Autodesk Fusion 360 part; units mm, degrees
(part 2 of 2)
sketch "Sketch23" plane through (0, 5, 0) normal (0, 1, 0) x (-1, 0, 0)
  circle A0 centre (-181.5, -92.25) radius 5
  circle A1 centre (-181.5, -115.25) radius 5
  circle A2 centre (-154.5, -126.75) radius 5
  circle A3 centre (-154.5, -103.75) radius 5
  circle A4 centre (-186.75, -72.25) radius 4
  circle A5 centre (-140.75, -72.25) radius 4
  circle A6 centre (-94.75, -72.25) radius 4
  circle A7 centre (-48.75, -72.25) radius 4
  circle A8 centre (-190, -170) radius 3.75
  circle A9 centre (-13.25, -72.25) radius 4
  circle A10 centre (-59.25, -72.25) radius 4
  circle A11 centre (-105.25, -72.25) radius 4
  circle A12 centre (-151.25, -72.25) radius 4
  circle A13 centre (-154.5, -92.25) radius 5
  circle A14 centre (-154.5, -115.25) radius 5
  circle A15 centre (-181.5, -126.75) radius 5
  circle A16 centre (-181.5, -103.75) radius 5
  line L0 (-116.5, -98) -> (-126.5, -98)
  line L1 (-126.5, -98) -> (-126.5, -88)
  line L2 (-126.5, -88) -> (-116.5, -88)
  line L3 (-116.5, -88) -> (-116.5, -98)
  line L4 (0, -101) -> (-8, -101)
  line L5 (-8, -101) -> (-8, -85)
  line L6 (-8, -85) -> (0, -85)
  line L7 (0, -85) -> (0, -67)
  line L8 (0, -67) -> (-8, -67)
  line L9 (-8, -67) -> (-8, -51)
  line L10 (-8, -51) -> (0, -51)
  line L11 (0, -51) -> (0, -11)
  line L12 (0, -11) -> (-6.3858, -11)
  arc A17 (-12.9938, -7.7418) -> (-6.3858, -11) centre (-10, -10) ccw
  arc A18 (-14.6419, 0) -> (-12.9938, -7.7418) centre (-13.25, -3.75) ccw
  line L13 (-14.6419, 0) -> (-47.3581, 0)
  arc A19 (-50.1419, 0) -> (-47.3581, 0) centre (-48.75, -3.75) ccw
  line L14 (-50.1419, 0) -> (-57.8581, 0)
  arc A20 (-60.6419, 0) -> (-57.8581, 0) centre (-59.25, -3.75) ccw
  line L15 (-60.6419, 0) -> (-93.3581, 0)
  arc A21 (-96.1419, 0) -> (-93.3581, 0) centre (-94.75, -3.75) ccw
  line L16 (-96.1419, 0) -> (-103.8581, 0)
  arc A22 (-106.6419, 0) -> (-103.8581, 0) centre (-105.25, -3.75) ccw
  line L17 (-106.6419, 0) -> (-139.3581, 0)
  arc A23 (-142.1419, 0) -> (-139.3581, 0) centre (-140.75, -3.75) ccw
  line L18 (-142.1419, 0) -> (-149.8581, 0)
  arc A24 (-152.6419, 0) -> (-149.8581, 0) centre (-151.25, -3.75) ccw
  line L19 (-152.6419, 0) -> (-185.3581, 0)
  arc A25 (-187.0062, -7.7418) -> (-185.3581, 0) centre (-186.75, -3.75) ccw
  arc A26 (-193.6142, -11) -> (-187.0062, -7.7418) centre (-190, -10) ccw
  line L20 (-193.6142, -11) -> (-200, -11)
  line L21 (-200, -11) -> (-200, -65)
  line L22 (-200, -65) -> (-192, -65)
  line L23 (-192, -65) -> (-192, -78)
  line L24 (-192, -78) -> (-200, -78)
  line L25 (-200, -78) -> (-200, -180)
  line L26 (-200, -180) -> (-180, -180)
  line L27 (-180, -180) -> (-180, -140)
  line L28 (-180, -140) -> (-124.5, -140)
  line L29 (-124.5, -140) -> (-124.5, -110)
  line L30 (-124.5, -110) -> (-55.5, -110)
  line L31 (-55.5, -110) -> (-55.5, -140)
  line L32 (-55.5, -140) -> (-8, -140)
  line L33 (-8, -140) -> (-8, -129)
  line L34 (-8, -129) -> (0, -129)
  line L35 (0, -129) -> (0, -101)
  line L36 (-55.5, -110) -> (-124.5, -110)
  line L37 (-124.5, -110) -> (-124.5, -115)
  line L38 (-124.5, -115) -> (-55.5, -115)
  line L39 (-55.5, -115) -> (-55.5, -110)
  dimension "d326_1" = 69
  dimension "d327_1" = 5
  constraint horizontal L36
  constraint vertical L37
  constraint horizontal L38
  constraint vertical L39
  constraint coincident L30.end L31.start
  measures "d326_1" distance of L30.end L29.end
  measures "d327_1" distance of L30.end L38.end
extrude "Extrude18" add sketch "Sketch23" along normal blind 11.5 separate body contours L29 L30 L31 L36 L37 L38 L39 makes body 3
combine "Combine1" operation cut target body 3 tool bodies 1 keep tools
sketch "Sketch24" plane through (0, 16.5, 0) normal (0, 1, 0) x (-1, 0, 0)
  line L0 (-119.5, -110) -> (-119.5, -115)
  line L1 (-119.5, -115) -> (-60.5, -115)
  line L2 (-60.5, -115) -> (-60.5, -110)
  line L3 (-60.5, -110) -> (-119.5, -110)
  line L4 (-119.5, -115) -> (-115.5, -115)
  line L5 (-115.5, -115) -> (-115.5, -119)
  line L6 (-115.5, -119) -> (-119.5, -119)
  line L7 (-119.5, -119) -> (-119.5, -115)
  dimension "d330_1" = 4
  dimension "d331_1" = 4
  constraint horizontal L4
  constraint vertical L5
  constraint horizontal L6
  constraint vertical L7
  constraint coincident L0.end L1.start
  measures "d330_1" distance of L0.end L4.end
  measures "d331_1" distance of L0.end L6.end
extrude "Extrude19" add sketch "Sketch24" against normal blind 5 contours L1 L4 L5 L6 L7 bodies 3
hole "Hole35" at (78.25, 10, -112.5) direction (0, -1, 0) diameter 2.5 end through all bodies 1
hole "Hole36" at (101.75, 10, -112.5) direction (0, -1, 0) diameter 2.5 end through all bodies 1
sketch "Sketch26" plane through (0, 10, 0) normal (0, 1, 0) x (-1, 0, 0)
  circle A0 centre (-78.25, -112.5) radius 1.25
  line L0 (-68.5, -115) -> (-68.5, -110)
  line L1 (-68.5, -110) -> (-88, -110)
  line L2 (-88, -110) -> (-88, -115)
  line L3 (-88, -115) -> (-68.5, -115)
  circle A1 centre (-78.25, -112.5) radius 1.5
  dimension "d341_1" = 3
  constraint concentric A0 A1
  measures "d341_1" diameter of A1
extrude "Extrude20" cut sketch "Sketch26" along normal up to surface (6.5 mm away) contours A0 | A1 bodies 3
sketch "Sketch27" plane through (0, 10, 0) normal (0, 1, 0) x (-1, 0, 0)
  circle A0 centre (-101.75, -112.5) radius 1.25
  line L0 (-92, -115) -> (-92, -110)
  line L1 (-92, -110) -> (-111.5, -110)
  line L2 (-111.5, -110) -> (-111.5, -115)
  line L3 (-111.5, -115) -> (-92, -115)
  circle A1 centre (-101.75, -112.5) radius 1.5
  dimension "d344_1" = 3
  constraint concentric A0 A1
  measures "d344_1" diameter of A1
extrude "Extrude21" cut sketch "Sketch27" along normal up to surface (6.5 mm away) contours A0 | A1 bodies 3
extrude "Extrude22" cut 1 faces at (60.5, 12.1667, -113.3333) along direction (1, 0, 0) blind 0.5 on bodies 3 bodies 3
extrude "Extrude23" cut 1 faces at (64.5, 9, -111.6667) along direction (1, 0, 0) blind 0.5 on bodies 3 bodies 3
extrude "Extrude24" cut 1 faces at (68.5, 9, -111.6667) along direction (-1, 0, 0) blind 0.5 on bodies 3 bodies 3
extrude "Extrude25" cut 1 faces at (88, 8, -111.6667) along direction (1, 0, 0) blind 0.5 on bodies 3 bodies 3
extrude "Extrude26" cut 1 faces at (92, 9, -111.6667) along direction (-1, 0, 0) blind 0.5 on bodies 3 bodies 3
extrude "Extrude27" cut 1 faces at (111.5, 9, -111.6667) along direction (1, 0, 0) blind 0.5 on bodies 3 bodies 3
extrude "Extrude28" cut 1 faces at (119.5, 11.6667, -111.6667) along direction (-1, 0, 0) blind 0.5 on bodies 3 bodies 3
extrude "Extrude29" cut 1 faces at (115.5, 14.8333, -116.3333) along direction (1, 0, 0) blind 0.5 on bodies 3 bodies 3
extrude "Extrude30" cut 1 faces at (117, 14.8333, -119) along direction (0, 0, 1) blind 0.5 on bodies 3 bodies 3
sketch "Sketch28" plane through (0, 75, 0) normal (0, 1, 0) x (-1, 0, 0)
  line L0 (-180, -145) -> (-5, -145)
  line L1 (-5, -145) -> (-5, -175)
  line L2 (-5, -175) -> (-180, -175)
  line L3 (-180, -175) -> (-180, -180)
  line L4 (-180, -180) -> (0, -180)
  line L5 (0, -180) -> (0, -140)
  line L6 (0, -140) -> (-180, -140)
  line L7 (-180, -140) -> (-180, -145)
  line L8 (0, -180) -> (-180, -180)
  line L9 (-180, -180) -> (-180, -140)
  line L10 (-180, -140) -> (0, -140)
  line L11 (0, -140) -> (0, -180)
  line L12 (-185.5, -134.5) -> (5.5, -134.5)
  line L13 (5.5, -134.5) -> (5.5, -185.5)
  line L14 (5.5, -185.5) -> (-185.5, -185.5)
  line L15 (-185.5, -185.5) -> (-185.5, -134.5)
  line L16 (-180.5, -139.5) -> (0.5, -139.5)
  line L17 (0.5, -139.5) -> (0.5, -180.5)
  line L18 (0.5, -180.5) -> (-180.5, -180.5)
  line L19 (-180.5, -180.5) -> (-180.5, -139.5)
  constraint horizontal L8
  constraint vertical L9
  constraint horizontal L10
  constraint vertical L11
  constraint coincident L6.end L7.start
  constraint coincident L4.end L5.start
extrude "Extrude33" add sketch "Sketch28" against normal blind 15 separate body contours L12 L13 L14 L15 makes body 4
extrude "Extrude34" add sketch "Sketch28" along normal blind 5 contours L0 L1 L2 L3 L4 L5 L6 L7 L8 L9 L10 L11 | L0 L1 L2 L9 | L12 L13 L14 L15 | L16 L17 L18 L19 bodies 4
sketch "Sketch29" plane through (0, 0, -140) normal (0, 0, 1) x (1, 0, 0)
  arc A0 (6, 7) -> (8, 5) centre (8, 7) ccw
  line L0 (8, 5) -> (55.5, 5)
  line L1 (55.5, 5) -> (55.5, 16.5)
  line L2 (55.5, 16.5) -> (118.5, 16.5)
  line L3 (118.5, 16.5) -> (118.5, 35)
  line L4 (118.5, 35) -> (124.5, 35)
  line L5 (124.5, 35) -> (124.5, 5)
  line L6 (124.5, 5) -> (180, 5)
  line L7 (180, 5) -> (180, 75)
  line L8 (180, 75) -> (0, 75)
  line L9 (0, 75) -> (0, 35)
  line L10 (0, 35) -> (6, 35)
  line L11 (6, 35) -> (6, 7)
  line L12 (180, 75) -> (170, 75)
  line L13 (170, 75) -> (170, 70)
  line L14 (170, 70) -> (180, 70)
  line L15 (180, 70) -> (180, 75)
  line L16 (170, 70) -> (165, 70)
  line L17 (165, 70) -> (165, 65)
  line L18 (165, 65) -> (170, 65)
  line L19 (170, 65) -> (170, 70)
  line L20 (0, 75) -> (10, 75)
  line L21 (10, 75) -> (10, 70)
  line L22 (10, 70) -> (0, 70)
  line L23 (0, 70) -> (0, 75)
  line L24 (10, 70) -> (15, 70)
  line L25 (15, 70) -> (15, 65)
  line L26 (15, 65) -> (10, 65)
  line L27 (10, 65) -> (10, 70)
  line L28 (165, 65) -> (170, 70)
  line L29 (15, 70) -> (10, 65)
  circle A1 centre (12.5, 67.5) radius 1.25
  circle A2 centre (167.5, 67.5) radius 1.25
  circle A3 centre (12.5, 67.5) radius 1.75
  circle A4 centre (167.5, 67.5) radius 1.75
  dimension "d377_1" = 10
  dimension "d378_1" = 5
  dimension "d379_1" = 5
  dimension "d380_1" = 5
  dimension "d381_1" = 10
  dimension "d382_1" = 5
  dimension "d383_1" = 5
  dimension "d384_1" = 5
  dimension "d385_1" = 2.5
  dimension "d386_1" = 2.5
  dimension "d399_1" = 3.5
  dimension "d400_1" = 3.5
  constraint horizontal L12
  constraint vertical L13
  constraint horizontal L14
  constraint vertical L15
  constraint coincident L7.end L8.start
  constraint horizontal L16
  constraint vertical L17
  constraint horizontal L18
  constraint vertical L19
  constraint horizontal L20
  constraint vertical L21
  constraint horizontal L22
  constraint vertical L23
  constraint coincident L8.end L9.start
  constraint horizontal L24
  constraint vertical L25
  constraint horizontal L26
  constraint vertical L27
  constraint midpoint L29 A1.centre
  constraint midpoint L28 A2.centre
  constraint concentric A1 A3
  constraint concentric A2 A4
  measures "d377_1" distance of L7.end L12.end
  measures "d378_1" distance of L7.end L14.end
  measures "d379_1" distance of L13.end L16.end
  measures "d380_1" distance of L13.end L18.end
  measures "d381_1" distance of L8.end L20.end
  measures "d382_1" distance of L8.end L22.end
  measures "d383_1" distance of L21.end L24.end
  measures "d384_1" distance of L21.end L26.end
  measures "d385_1" diameter of A1
  measures "d386_1" diameter of A2
  measures "d399_1" diameter of A3
  measures "d400_1" diameter of A4
extrude "Extrude35" cut sketch "Sketch29" against normal up to surface (5 mm away) contours L29 A1 | L29 A1 | L28 A2 | L28 A2 bodies 1
sketch "Sketch30" plane through (0, 0, 0) normal (-1, 0, 0) x (0, 0, 1)
  line L0 (-180, 0) -> (0, 0)
  line L1 (0, 0) -> (0, 35)
  line L2 (0, 35) -> (-6, 35)
  line L3 (-6, 35) -> (-6, 10)
  arc A0 (-11, 5) -> (-6, 10) centre (-11, 10) ccw
  line L4 (-11, 5) -> (-51, 5)
  arc A1 (-56, 10) -> (-51, 5) centre (-51, 10) ccw
  line L5 (-56, 10) -> (-56, 35)
  line L6 (-56, 35) -> (-62, 35)
  line L7 (-62, 35) -> (-62, 10)
  arc A2 (-67, 5) -> (-62, 10) centre (-67, 10) ccw
  line L8 (-67, 5) -> (-85, 5)
  arc A3 (-90, 10) -> (-85, 5) centre (-85, 10) ccw
  line L9 (-90, 10) -> (-90, 35)
  line L10 (-90, 35) -> (-96, 35)
  line L11 (-96, 35) -> (-96, 10)
  arc A4 (-101, 5) -> (-96, 10) centre (-101, 10) ccw
  line L12 (-101, 5) -> (-129, 5)
  arc A5 (-134, 10) -> (-129, 5) centre (-129, 10) ccw
  line L13 (-134, 10) -> (-134, 35)
  line L14 (-134, 35) -> (-140, 35)
  line L15 (-140, 35) -> (-140, 75)
  line L16 (-140, 75) -> (-180, 75)
  line L17 (-180, 75) -> (-180, 0)
  line L18 (-180, 75) -> (-140, 75)
  line L19 (-140, 75) -> (-140, 70)
  line L20 (-140, 70) -> (-180, 70)
  line L21 (-180, 70) -> (-180, 75)
  line L22 (-160, 75) -> (-160, 70)
  line L23 (-160, 70) -> (-162.5, 70)
  line L24 (-162.5, 70) -> (-162.5, 65)
  line L25 (-162.5, 65) -> (-160, 65)
  line L26 (-160, 65) -> (-160, 70)
  line L27 (-160, 70) -> (-157.5, 70)
  line L28 (-157.5, 70) -> (-157.5, 65)
  line L29 (-157.5, 65) -> (-160, 65)
  line L30 (-160, 65) -> (-160, 70)
  circle A6 centre (-160, 67.5) radius 1.25
  circle A7 centre (-160, 67.5) radius 1.75
  dimension "d389_1" = 40
  dimension "d390_1" = 5
  dimension "d391_1" = 2.5
  dimension "d392_1" = 5
  dimension "d393_1" = 2.5
  dimension "d394_1" = 5
  dimension "d395_1" = 2.5
  dimension "d401_1" = 3.5
  constraint horizontal L18
  constraint vertical L19
  constraint horizontal L20
  constraint vertical L21
  constraint coincident L16.end L17.start
  constraint midpoint L18 L22.start
  constraint midpoint L20 L22.end
  constraint horizontal L23
  constraint vertical L24
  constraint horizontal L25
  constraint vertical L26
  constraint horizontal L27
  constraint vertical L28
  constraint horizontal L29
  constraint vertical L30
  constraint midpoint L26 A6.centre
  constraint concentric A6 A7
  measures "d389_1" distance of L16.end L15.end
  measures "d390_1" distance of L16.end L20.end
  measures "d391_1" distance of L22.end L23.end
  measures "d392_1" distance of L22.end L25.end
  measures "d393_1" distance of L22.end L27.end
  measures "d394_1" distance of L22.end L25.end
  measures "d395_1" diameter of A6
  measures "d401_1" diameter of A7
extrude "Extrude36" cut sketch "Sketch30" against normal up to surface (5 mm away) contours L26 L30 A6 | L26 L30 A6 bodies 1
extrude "Extrude37" cut sketch "Sketch29" along normal up to surface (5.5 mm away) contours L29 A1 A3 | L29 A1 A3 | L29 A1 | L29 A1 | L28 A2 A4 | L28 A2 A4 | L28 A2 | L28 A2 bodies 4
extrude "Extrude38" cut sketch "Sketch30" along normal up to surface (5.5 mm away) contours L26 L30 A6 A7 | L26 L30 A6 A7 | L26 L30 A6 | L26 L30 A6 bodies 4
sketch "Sketch31" plane through (185.5, 0, 0) normal (1, 0, 0) x (0, 0, -1)
  line L0 (134.5, 80) -> (134.5, 60)
  line L1 (134.5, 60) -> (185.5, 60)
  line L2 (185.5, 60) -> (185.5, 80)
  line L3 (185.5, 80) -> (134.5, 80)
  line L4 (134.5, 80) -> (185.5, 80)
  line L5 (185.5, 80) -> (185.5, 75)
  line L6 (185.5, 75) -> (134.5, 75)
  line L7 (134.5, 75) -> (134.5, 80)
  line L8 (134.5, 75) -> (140, 75)
  line L9 (140, 75) -> (140, 60)
  line L10 (140, 60) -> (134.5, 60)
  line L11 (134.5, 60) -> (134.5, 75)
  line L12 (185.5, 75) -> (180, 75)
  line L13 (180, 75) -> (180, 60)
  line L14 (180, 60) -> (185.5, 60)
  line L15 (185.5, 60) -> (185.5, 75)
  line L16 (140, 75) -> (145, 75)
  line L17 (145, 75) -> (145, 60)
  line L18 (145, 60) -> (140, 60)
  line L19 (140, 60) -> (140, 75)
  line L20 (180, 75) -> (175, 75)
  line L21 (175, 75) -> (175, 60)
  line L22 (175, 60) -> (180, 60)
  line L23 (180, 60) -> (180, 75)
  dimension "d406_1" = 5
  dimension "d407_1" = 5.5
  dimension "d408_1" = 5.5
  dimension "d409_1" = 5
  dimension "d410_1" = 5
  constraint horizontal L4
  constraint vertical L5
  constraint horizontal L6
  constraint vertical L7
  constraint coincident L0.start L3.end
  constraint collinear L2 L5
  constraint horizontal L8
  constraint vertical L9
  constraint horizontal L10
  constraint vertical L11
  constraint collinear L1 L10
  constraint horizontal L12
  constraint vertical L13
  constraint horizontal L14
  constraint vertical L15
  constraint collinear L1 L14
  constraint horizontal L16
  constraint vertical L17
  constraint horizontal L18
  constraint vertical L19
  constraint horizontal L20
  constraint vertical L21
  constraint horizontal L22
  constraint vertical L23
  constraint collinear L1 L18
  constraint collinear L1 L22
  measures "d406_1" distance of L0.start L6.end
  measures "d407_1" distance of L6.end L8.end
  measures "d408_1" distance of L5.end L12.end
  measures "d409_1" distance of L8.end L16.end
  measures "d410_1" distance of L12.end L20.end
extrude "Extrude39" cut sketch "Sketch31" against normal up to surface (5 mm away) contours L1 L6 L17 L21 bodies 4
sketch "Sketch32" plane through (0, 40, 0) normal (0, 1, 0) x (-1, 0, 0)
  circle A0 centre (-3, -3) radius 1.75
  circle A1 centre (-121.5, -137) radius 1.75
  circle A2 centre (-121.5, -93) radius 1.75
  circle A3 centre (-197, -3) radius 1.75
  circle A4 centre (-3, -59) radius 1.75
  circle A5 centre (-3, -137) radius 1.75
  circle A6 centre (-3, -93) radius 1.75
  circle A7 centre (-197, -73) radius 1.75
  line L0 (-124.5, -140) -> (0, -140)
  line L1 (0, -140) -> (0, 0)
  line L2 (0, 0) -> (-200, 0)
  line L3 (-200, 0) -> (-200, -76)
  line L4 (-200, -76) -> (-124.5, -76)
  line L5 (-124.5, -76) -> (-124.5, -140)
  line L6 (-100, 0) -> (-100, -140)
  circle A8 centre (-100, 0) radius 10
  circle A9 centre (-100, -35) radius 10
  circle A10 centre (-100, -70) radius 10
  circle A11 centre (-100, -105) radius 10
  circle A12 centre (-100, -140) radius 10
  line L7 (-21.5, -113) -> (-78.5, -113)
  line L8 (-78.5, -113) -> (-78.5, 0)
  line L9 (-78.5, 0) -> (-21.5, 0)
  line L10 (-21.5, 0) -> (-21.5, -113)
  line L11 (-21.5, -113) -> (-78.5, 0) construction
  line L12 (-78.5, -113) -> (-21.5, 0) construction
  line L13 (-25.5, -4) -> (-25.5, -109)
  line L14 (-25.5, -109) -> (-74.5, -109)
  line L15 (-74.5, -109) -> (-74.5, -4)
  line L16 (-74.5, -4) -> (-25.5, -4)
  circle A13 centre (-74.5, -109) radius 3
  circle A14 centre (-25.5, -109) radius 3
  line L17 (-78.5, 0) -> (-69.25, 0)
  line L18 (-69.25, 0) -> (-69.25, -113)
  line L19 (-69.25, -113) -> (-78.5, -113)
  line L20 (-78.5, -113) -> (-78.5, 0)
  line L21 (-21.5, 0) -> (-30.75, 0)
  line L22 (-30.75, 0) -> (-30.75, -113)
  line L23 (-30.75, -113) -> (-21.5, -113)
  line L24 (-21.5, -113) -> (-21.5, 0)
  line L25 (-78.5, -113) -> (-21.5, -113)
  line L26 (-21.5, -113) -> (-21.5, -46.5)
  line L27 (-21.5, -46.5) -> (-78.5, -46.5)
  line L28 (-78.5, -46.5) -> (-78.5, -113)
  circle A15 centre (-30.75, -46.5) radius 3
  circle A16 centre (-69.25, -46.5) radius 3
  line L29 (-78.5, 0) -> (-21.5, 0)
  line L30 (-21.5, 0) -> (-21.5, -13.75)
  line L31 (-21.5, -13.75) -> (-78.5, -13.75)
  line L32 (-78.5, -13.75) -> (-78.5, 0)
  line L33 (-78.5, 0) -> (-74.5, 0)
  line L34 (-74.5, 0) -> (-74.5, -6)
  line L35 (-74.5, -6) -> (-78.5, -6)
  line L36 (-78.5, -6) -> (-78.5, 0)
  line L37 (-21.5, -13.75) -> (-25.5, -13.75)
  line L38 (-25.5, -13.75) -> (-25.5, -19.75)
  line L39 (-25.5, -19.75) -> (-21.5, -19.75)
  line L40 (-21.5, -19.75) -> (-21.5, -13.75)
  line L41 (-74.5, 0) -> (-72.5, 0)
  line L42 (-72.5, 0) -> (-72.5, -4)
  line L43 (-72.5, -4) -> (-74.5, -4)
  line L44 (-74.5, -4) -> (-74.5, 0)
  point P0 (-50, -56.5)
  dimension "d415_1" = 20
  dimension "d418_1" = 140
  dimension "d419_1" = 0
  dimension "d420_1" = 57
  dimension "d421_1" = 113
  dimension "d422_1" = 4
  dimension "d423_1" = 6
  dimension "d424_1" = 6
  dimension "d425_1" = 9.25
  dimension "d426_1" = 9.25
  dimension "d427_1" = 66.5
  dimension "d428_1" = 6
  dimension "d429_1" = 6
  dimension "d430_1" = 57
  dimension "d431_1" = 13.75
  dimension "d432_1" = 4
  dimension "d433_1" = 6
  dimension "d434_1" = 4
  dimension "d435_1" = 6
  dimension "d440_1" = 2
  dimension "d441_1" = 4
  constraint midpoint L2 L6.start
  constraint coincident L0 L6.end
  constraint perpendicular L0 L6
  constraint coincident L6.start A8.centre
  constraint horizontal L7
  constraint perpendicular L7 L8
  constraint parallel L7 L9
  constraint parallel L8 L10
  constraint coincident L11 P0
  constraint coincident L12 P0
  constraint coincident L14.end L15.start
  constraint coincident L13.end L14.start
  constraint horizontal L17
  constraint vertical L18
  constraint horizontal L19
  constraint vertical L20
  constraint horizontal L21
  constraint vertical L22
  constraint horizontal L23
  constraint vertical L24
  constraint collinear L7 L23
  constraint collinear L7 L19
  constraint horizontal L25
  constraint vertical L26
  constraint horizontal L27
  constraint vertical L28
  constraint coincident L22 A15.centre
  constraint coincident L27 A15.centre
  constraint coincident L27 A16.centre
  constraint coincident L18 A16.centre
  constraint coincident L7.start L26
  constraint horizontal L29
  constraint vertical L30
  constraint horizontal L31
  constraint vertical L32
  constraint horizontal L33
  constraint vertical L34
  constraint horizontal L35
  constraint vertical L36
  constraint horizontal L37
  constraint vertical L38
  constraint horizontal L39
  constraint vertical L40
  constraint horizontal L41
  constraint vertical L42
  constraint horizontal L43
  constraint vertical L44
  constraint collinear L2 L29
  measures "d415_1" diameter of A8
  measures "d420_1" distance of L8.end L9.end
  measures "d421_1" distance of L7.end L8.end
  measures "d423_1" diameter of A13
  measures "d424_1" diameter of A14
  measures "d425_1" distance of L8.end L17.end
  measures "d426_1" distance of L9.end L21.end
  measures "d427_1" distance of L7.end L27.end
  measures "d428_1" diameter of A15
  measures "d429_1" diameter of A16
  measures "d430_1" distance of L8.end L9.end
  measures "d431_1" distance of L8.end L31.end
  measures "d432_1" distance of L8.end L33.end
  measures "d433_1" distance of L8.end L35.end
  measures "d434_1" distance of L30.end L37.end
  measures "d435_1" distance of L30.end L39.end
  measures "d440_1" distance of L33.end L41.end
  measures "d441_1" distance of L33.end L15.end
extrude "Extrude40" add sketch "Sketch32" along normal blind 5 contours L10 L13 L24 L31 L37 L38 L39 L40 | L2 L9 L16 L17 L29 L34 L41 L42 L43 L44 | L2 L8 L9 L15 L17 L20 L29 L32 L33 L34 L35 L36 L44 | L22 L27 A15 | L22 L27 A15 | L18 L27 A16 | L18 L27 A16 | L22 L27 A15 | L22 L27 A15 | L13 L14 A14 | L13 L14 A14 | L18 L27 A16 | L18 L27 A16 | L14 L15 A13 | L14 L15 A13 bodies 2
extrude "Extrude41" add 2 faces at (22.8333, 45, -17.75) (77.1667, 45, -3.3333) along direction (0, 1, 0) blind 1 on bodies 2 bodies 2
hole "Hole37" at (69.25, 45, -46.5) direction (0, -1, 0) diameter 2.5 end up to surface (10 mm away) bodies 2
hole "Hole38" at (30.75, 45, -46.5) direction (0, -1, 0) diameter 2.5 end up to surface (10 mm away) bodies 2
hole "Hole39" at (74.5, 45, -109) direction (0, -1, 0) diameter 2.5 end up to surface (10 mm away) bodies 2
hole "Hole40" at (25.5, 45, -109) direction (0, -1, 0) diameter 2.5 end up to surface (10 mm away) bodies 2
fillet "Fillet5" radius 2 8 edges at (28.297, 40, -107.9152) (77.297, 40, -107.9152) (33.547, 40, -45.4152) (72.047, 40, -45.4152) (23.5, 40, -13.75) (21.5, 40, -16.75) (25.5, 40, -16.75) (23.5, 40, -19.75) on bodies 2
fillet "Fillet5" radius 2 3 edges at (78.5, 40, -3) (76.5, 40, -6) (72.5, 40, -2) on bodies 2
fillet "Fillet6" radius 2 2 edges at (74.5, 40, -5) (73.5, 40, -4) on bodies 2
extrude "Extrude42" cut sketch "Sketch32" against normal up to surface (5 mm away) contours L6 A11 | L6 A11 | L6 A10 | L6 A10 | L6 A9 | L6 A9 bodies 2
sketch "Sketch33" plane through (0, 16.5, 0) normal (0, 1, 0) x (-1, 0, 0)
  circle A0 centre (-101.75, -112.5) radius 1.5
  circle A1 centre (-78.25, -112.5) radius 1.5
  line L0 (-119, -110) -> (-119, -118.5)
  line L1 (-119, -118.5) -> (-116, -118.5)
  line L2 (-116, -118.5) -> (-116, -115)
  line L3 (-61, -115) -> (-61, -110)
  circle A2 centre (-78.25, -112.5) radius 3.25
  circle A3 centre (-101.75, -112.5) radius 3.25
  line L4 (-61, -110) -> (-119, -110)
  line L5 (-116, -115) -> (-61, -115)
  point P0 (-78.25, -112.5)
  point P1 (-101.75, -112.5)
  dimension "d468_1" = 6.5
  dimension "d469_1" = 6.5
  constraint coincident P0 A1.centre
  constraint coincident A0.centre A3.centre
  constraint coincident P1 A0.centre
  measures "d468_1" diameter of A2
  measures "d469_1" diameter of A3
extrude "Extrude43" cut sketch "Sketch33" against normal blind 2.5 contours A3 L4 L5 | A3 L4 | A3 L5 | A2 L4 L5 | A2 L4 | A2 L5 bodies 3
sketch "Sketch34" plane through (0, 0, -134.5) normal (0, 0, 1) x (1, 0, 0)
  circle A0 centre (167.5, 67.5) radius 1.75
  circle A1 centre (12.5, 67.5) radius 1.75
  line L0 (-5.5, 80) -> (-5.5, 60)
  line L1 (-5.5, 60) -> (185.5, 60)
  line L2 (185.5, 60) -> (185.5, 80)
  line L3 (185.5, 80) -> (-5.5, 80)
  circle A2 centre (12.5, 67.5) radius 3.25
  circle A3 centre (167.5, 67.5) radius 3.25
  dimension "d470_1" = 6.5
  dimension "d471_1" = 6.5
  constraint concentric A1 A2
  constraint concentric A0 A3
  measures "d470_1" diameter of A2
  measures "d471_1" diameter of A3
extrude "Extrude44" cut sketch "Sketch34" against normal blind 2.5 contours A2 | A3 bodies 4
sketch "Sketch35" plane through (-5.5, 0, 0) normal (-1, 0, 0) x (0, 0, 1)
  circle A0 centre (-160, 67.5) radius 1.75
  line L0 (-185.5, 80) -> (-185.5, 60)
  line L1 (-185.5, 60) -> (-134.5, 60)
  line L2 (-134.5, 60) -> (-134.5, 80)
  line L3 (-134.5, 80) -> (-185.5, 80)
  circle A1 centre (-160, 67.5) radius 3.25
  dimension "d474_1" = 6.5
  constraint concentric A0 A1
  measures "d474_1" diameter of A1
extrude "Extrude45" cut sketch "Sketch35" against normal blind 2.5 contours A1 bodies 4
sketch "Sketch36" plane through (0, 40, 0) normal (0, 1, 0) x (-1, 0, 0)
  circle A0 centre (-100, -105) radius 10
  circle A1 centre (-100, -70) radius 10
  circle A2 centre (-100, -35) radius 10
  circle A3 centre (-74.5, -109) radius 5
  circle A4 centre (-30.75, -46.5) radius 5
  circle A5 centre (-3, -3) radius 1.75
  circle A6 centre (-121.5, -137) radius 1.75
  circle A7 centre (-121.5, -93) radius 1.75
  circle A8 centre (-197, -3) radius 1.75
  circle A9 centre (-3, -59) radius 1.75
  circle A10 centre (-3, -137) radius 1.75
  circle A11 centre (-3, -93) radius 1.75
  circle A12 centre (-197, -73) radius 1.75
  line L0 (-124.5, -140) -> (0, -140)
  line L1 (0, -140) -> (0, 0)
  line L2 (-80.5, 0) -> (-200, 0)
  line L3 (-200, 0) -> (-200, -76)
  line L4 (-200, -76) -> (-124.5, -76)
  line L5 (-124.5, -76) -> (-124.5, -140)
  line L6 (-19.5, -21.75) -> (-27.5, -21.75)
  line L7 (-27.5, -21.75) -> (-27.5, -11.75)
  line L8 (-27.5, -11.75) -> (-19.5, -11.75)
  line L9 (-19.5, -11.75) -> (-19.5, -21.75)
  circle A13 centre (-25.5, -109) radius 5
  circle A14 centre (-69.25, -46.5) radius 5
  line L10 (0.25, -140.25) -> (-6.25, -140.25)
  line L11 (-6.25, -140.25) -> (-6.25, -133.75)
  line L12 (-6.25, -133.75) -> (0.25, -133.75)
  line L13 (0.25, -133.75) -> (0.25, -140.25)
  line L14 (0.25, -140.25) -> (-6.25, -133.75) construction
  line L15 (-6.25, -140.25) -> (0.25, -133.75) construction
  line L16 (0.25, -6.25) -> (-6.25, -6.25)
  line L17 (-6.25, -6.25) -> (-6.25, 0.25)
  line L18 (-6.25, 0.25) -> (0.25, 0.25)
  line L19 (0.25, 0.25) -> (0.25, -6.25)
  line L20 (0.25, -6.25) -> (-6.25, 0.25) construction
  line L21 (-6.25, -6.25) -> (0.25, 0.25) construction
  line L22 (-200.25, -6.25) -> (-193.75, -6.25)
  line L23 (-193.75, -6.25) -> (-193.75, 0.25)
  line L24 (-193.75, 0.25) -> (-200.25, 0.25)
  line L25 (-200.25, 0.25) -> (-200.25, -6.25)
  line L26 (-200.25, -6.25) -> (-193.75, 0.25) construction
  line L27 (-193.75, -6.25) -> (-200.25, 0.25) construction
  line L28 (-200.25, -76.25) -> (-193.75, -76.25)
  line L29 (-193.75, -76.25) -> (-193.75, -69.75)
  line L30 (-193.75, -69.75) -> (-200.25, -69.75)
  line L31 (-200.25, -69.75) -> (-200.25, -76.25)
  line L32 (-200.25, -76.25) -> (-193.75, -69.75) construction
  line L33 (-193.75, -76.25) -> (-200.25, -69.75) construction
  line L34 (-118.25, -140.25) -> (-124.75, -140.25)
  line L35 (-124.75, -140.25) -> (-124.75, -133.75)
  line L36 (-124.75, -133.75) -> (-118.25, -133.75)
  line L37 (-118.25, -133.75) -> (-118.25, -140.25)
  line L38 (-118.25, -140.25) -> (-124.75, -133.75) construction
  line L39 (-124.75, -140.25) -> (-118.25, -133.75) construction
  circle A15 centre (-121.5, -93) radius 3.25
  circle A16 centre (-3, -93) radius 3.25
  circle A17 centre (-3, -59) radius 3.25
  line L40 (-70.5, 0) -> (-70.5, -6)
  line L41 (-70.5, -6) -> (-72.5, -6)
  line L42 (-72.5, -6) -> (-72.5, -8)
  line L43 (-72.5, -8) -> (-80.5, -8)
  line L44 (-80.5, -8) -> (-80.5, 0)
  line L45 (0, 0) -> (-70.5, 0)
  point P0 (-3, -137)
  point P1 (-3, -3)
  point P2 (-197, -3)
  point P3 (-197, -73)
  point P4 (-121.5, -137)
  dimension "d477_1" = 6.5
  dimension "d478_1" = 6.5
  dimension "d479_1" = 6.5
  dimension "d480_1" = 6.5
  dimension "d481_1" = 6.5
  dimension "d482_1" = 6.5
  dimension "d483_1" = 6.5
  dimension "d484_1" = 6.5
  dimension "d485_1" = 6.5
  dimension "d486_1" = 6.5
  dimension "d487_1" = 6.5
  dimension "d488_1" = 6.5
  dimension "d489_1" = 6.5
  constraint horizontal L10
  constraint perpendicular L10 L11
  constraint parallel L10 L12
  constraint parallel L11 L13
  constraint coincident L14 P0
  constraint coincident L15 P0
  constraint coincident P0 A10.centre
  constraint horizontal L16
  constraint perpendicular L16 L17
  constraint parallel L16 L18
  constraint parallel L17 L19
  constraint coincident L20 P1
  constraint coincident L21 P1
  constraint coincident P1 A5.centre
  constraint horizontal L22
  constraint perpendicular L22 L23
  constraint parallel L22 L24
  constraint parallel L23 L25
  constraint coincident L26 P2
  constraint coincident L27 P2
  constraint coincident P2 A8.centre
  constraint horizontal L28
  constraint perpendicular L28 L29
  constraint parallel L28 L30
  constraint parallel L29 L31
  constraint coincident L32 P3
  constraint coincident L33 P3
  constraint coincident P3 A12.centre
  constraint horizontal L34
  constraint perpendicular L34 L35
  constraint parallel L34 L36
  constraint parallel L35 L37
  constraint coincident L38 P4
  constraint coincident L39 P4
  constraint coincident P4 A6.centre
  constraint concentric A7 A15
  constraint concentric A11 A16
  constraint concentric A9 A17
  measures "d477_1" distance of L11.end L12.end
  measures "d478_1" distance of L10.end L11.end
  measures "d479_1" distance of L17.end L18.end
  measures "d480_1" distance of L16.end L17.end
  measures "d481_1" distance of L23.end L24.end
  measures "d482_1" distance of L22.end L23.end
  measures "d483_1" distance of L29.end L30.end
  measures "d484_1" distance of L28.end L29.end
  measures "d485_1" distance of L35.end L36.end
  measures "d486_1" distance of L34.end L35.end
  measures "d487_1" diameter of A15
  measures "d488_1" diameter of A16
  measures "d489_1" diameter of A17
extrude "Extrude46" cut sketch "Sketch36" against normal blind 2.5 contours L0 L5 L36 L37 | L0 L1 L11 L12 | L5 A15 | L1 A16 | L3 L4 L29 L30 | L1 A17 | L2 L3 L22 L23 | L1 L16 L17 L45 picked at (-124.0833, -93) picked at (-0.4167, -93) picked at (-0.4167, -59) bodies 2
extrude "Extrude47" cut 1 faces at (121.1667, 12.1667, -119) along direction (0, 0, 1) up to surface (9 mm away) on bodies 1 bodies 1
extrude "Extrude48" cut 1 faces at (65, 9, -111.6667) along direction (1, 0, 0) up to surface (54 mm away) on bodies 3 bodies 3
extrude "Extrude49" cut 2 faces at (89.3333, 7, -111.6667) (67.1667, 7, -111.6667) along direction (0, 1, 0) up to surface end surface through (0, 5, 0) normal (0, 1, 0) offset 0 on bodies 1 bodies 1
extrude "Extrude50" cut 1 faces at (68.5, 8.3333, -111.6667) along direction (1, 0, 0) blind 6.5 on bodies 1 bodies 1
extrude "Extrude51" cut 1 faces at (88, 8.3333, -111.6667) along direction (-1, 0, 0) blind 6.5 on bodies 1 bodies 1
extrude "Extrude52" cut 1 faces at (92, 6.6667, -113.3333) along direction (1, 0, 0) blind 6.5 on bodies 1 bodies 1
sketch "Sketch37" plane through (0, 7, 0) normal (0, 1, 0) x (-1, 0, 0)
  line L0 (-115.5, -115) -> (-111.5, -115)
  line L1 (-111.5, -115) -> (-111.5, -110)
  line L2 (-111.5, -110) -> (-119.5, -110)
  line L3 (-119.5, -110) -> (-119.5, -119)
  line L4 (-119.5, -119) -> (-115.5, -119)
  line L5 (-115.5, -119) -> (-115.5, -115)
  line L6 (-111.5, -115) -> (-115.5, -115)
  line L7 (-115.5, -115) -> (-115.5, -110)
  line L8 (-115.5, -110) -> (-111.5, -110)
  line L9 (-111.5, -110) -> (-111.5, -115)
  constraint horizontal L6
  constraint vertical L7
  constraint horizontal L8
  constraint vertical L9
  constraint midpoint L2 L7.end
  constraint coincident L0.end L1.start
extrude "Extrude53" cut sketch "Sketch37" against normal up to surface (2 mm away) contours L0 L1 L2 L6 L7 L8 L9 bodies 1
extrude "Extrude54" cut 1 faces at (111.5, 6.6667, -111.6667) along direction (-1, 0, 0) blind 6.5 on bodies 1 bodies 1
extrude "Extrude55" cut 1 faces at (64.5, 8.3333, -111.6667) along direction (-1, 0, 0) up to surface (3 mm away) on bodies 1 bodies 1
sketch "Sketch38" plane through (0, 40, 0) normal (0, 1, 0) x (-1, 0, 0)
  circle A0 centre (-69.25, -46.5) radius 5
  circle A1 centre (-74.5, -109) radius 5
  circle A2 centre (-25.5, -109) radius 5
  circle A3 centre (-30.75, -46.5) radius 5
  line L0 (-19.5, -21.75) -> (-27.5, -21.75)
  line L1 (-27.5, -21.75) -> (-27.5, -11.75)
  line L2 (-27.5, -11.75) -> (-19.5, -11.75)
  line L3 (-19.5, -11.75) -> (-19.5, -21.75)
  circle A4 centre (-100, -35) radius 10
  circle A5 centre (-100, -70) radius 10
  circle A6 centre (-100, -105) radius 10
  line L4 (0, -6.25) -> (-6.25, -6.25)
  line L5 (-6.25, -6.25) -> (-6.25, 0)
  line L6 (-6.25, 0) -> (-70.5, 0)
  line L7 (-70.5, 0) -> (-70.5, -6)
  line L8 (-70.5, -6) -> (-72.5, -6)
  line L9 (-72.5, -6) -> (-72.5, -8)
  line L10 (-72.5, -8) -> (-80.5, -8)
  line L11 (-80.5, -8) -> (-80.5, 0)
  line L12 (-80.5, 0) -> (-193.75, 0)
  line L13 (-193.75, 0) -> (-193.75, -6.25)
  line L14 (-193.75, -6.25) -> (-200, -6.25)
  line L15 (-200, -6.25) -> (-200, -69.75)
  line L16 (-200, -69.75) -> (-193.75, -69.75)
  line L17 (-193.75, -69.75) -> (-193.75, -76)
  line L18 (-193.75, -76) -> (-124.5, -76)
  line L19 (-124.5, -76) -> (-124.5, -91.75)
  arc A7 (-124.5, -94.25) -> (-124.5, -91.75) centre (-121.5, -93) ccw
  line L20 (-124.5, -94.25) -> (-124.5, -133.75)
  line L21 (-124.5, -133.75) -> (-118.25, -133.75)
  line L22 (-118.25, -133.75) -> (-118.25, -140)
  line L23 (-118.25, -140) -> (-6.25, -140)
  line L24 (-6.25, -140) -> (-6.25, -133.75)
  line L25 (-6.25, -133.75) -> (0, -133.75)
  line L26 (0, -133.75) -> (0, -94.25)
  arc A8 (0, -91.75) -> (0, -94.25) centre (-3, -93) ccw
  line L27 (0, -91.75) -> (0, -60.25)
  arc A9 (0, -57.75) -> (0, -60.25) centre (-3, -59) ccw
  line L28 (0, -57.75) -> (0, -6.25)
  line L29 (-159.125, -76) -> (-159.125, 0) construction
  line L30 (-185.625, -56.5) -> (-132.625, -56.5) construction
  line L31 (-132.625, -56.5) -> (-132.625, -19.5) construction
  line L32 (-132.625, -19.5) -> (-185.625, -19.5) construction
  line L33 (-185.625, -19.5) -> (-185.625, -56.5) construction
  line L34 (-185.625, -56.5) -> (-132.625, -19.5) construction
  line L35 (-132.625, -56.5) -> (-185.625, -19.5) construction
  circle A10 centre (-132.625, -56.5) radius 1.25
  circle A11 centre (-132.625, -56.5) radius 3
  circle A12 centre (-185.625, -56.5) radius 3
  circle A13 centre (-185.625, -56.5) radius 1.25
  circle A14 centre (-185.625, -19.5) radius 3
  circle A15 centre (-185.625, -19.5) radius 1.25
  circle A16 centre (-132.625, -19.5) radius 3
  circle A17 centre (-132.625, -19.5) radius 1.25
  point P0 (-159.125, -38)
  dimension "d514_1" = 53
  dimension "d515_1" = 37
  dimension "d516_1" = 2.5
  dimension "d517_1" = 6
  constraint midpoint L18 L29.start
  constraint coincident L12 L29.end
  constraint perpendicular L12 L29
  constraint horizontal L30
  constraint perpendicular L30 L31
  constraint parallel L30 L32
  constraint parallel L31 L33
  constraint coincident L34 P0
  constraint coincident L35 P0
  constraint midpoint L29 P0
  constraint coincident L30.end L31.start
  constraint concentric A10 A11
  constraint coincident L30.start L33.end
  constraint concentric A12 A13
  constraint coincident L32.end L33.start
  constraint concentric A14 A15
  constraint coincident L31.end L32.start
  constraint concentric A16 A17
  constraint equal A10 A13
  constraint equal A10 A15
  constraint equal A10 A17
  constraint equal A11 A16
  constraint equal A11 A14
  constraint equal A11 A12
  measures "d514_1" distance of L31.end L32.end
  measures "d515_1" distance of L30.end L31.end
  measures "d516_1" diameter of A10
  measures "d517_1" diameter of A11
extrude "Extrude56" add sketch "Sketch38" along normal up to surface (5 mm away) contours A11 | A12 | A14 | A16 bodies 2
fillet "Fillet7" radius 2 4 edges at (135.422, 40, -55.4152) (135.422, 40, -18.4152) (188.422, 40, -55.4152) (188.422, 40, -18.4152) on bodies 2
extrude "Extrude57" cut 4 faces at (132.9471, 40, -56.1742) (185.9471, 40, -56.1742) (132.3196, 40, -19.0924) (185.3196, 40, -19.0924) along direction (0, 1, 0) up to surface end surface through (0, 35, 0) normal (0, -1, 0) offset 0 on bodies 2 bodies 2
hidden bodies 4
equation "d3_1 = width"
equation "d4_1 = length"
equation "d6_1 = height"
equation "d12_1 = -screw_offset"
equation "d19_2 = ( screw_head_diam - screw_hole_diam ) / 2"
equation "d20_2 = height"
equation "d25_1 = batt_width + batt_wall * 2"
equation "d26_2 = batt_length + batt_wall * 2"
equation "d27_2 = batt_wall"
equation "d28_2 = batt_height"
equation "d32_1 = -batt_pwr_height"
equation "d34_2 = batt_wall"
equation "d35_2 = batt_cel_length"
equation "d37_2 = -batt_cel_height"
equation "d46_2 = driver_space / 2"
equation "d47_2 = driver_length"
equation "d48_2 = driver_width"
equation "d49_2 = driver_length"
equation "d50_2 = driver_space"
equation "d51_2 = driver_length"
equation "d52_2 = driver_width"
equation "d53_2 = driver_length"
equation "d54_2 = driver_screw_offset"
equation "d55_2 = driver_screw_offset"
equation "d64_2 = elem_fix_spacer_height"
equation "d67_2 = driver_fix_fillet"
equation "d78_1 = ( batt_width + batt_wall * 2 ) / 2 - ( bms_width + bms_wall * 2 ) / 2"
equation "d79_1 = bms_length + bms_wall * 2"
equation "d81_1 = bms_width + bms_wall * 2"
equation "d82_1 = bms_length + bms_wall * 2"
equation "d83_1 = bms_wall"
equation "d91 = bms_thick + bms_wall * 2"
equation "d93 = bms_wall"
equation "d95_1 = bms_thick + slack_print"
equation "d109 = bms_bottom_slack"
equation "d111_1 = bms_bottom_slack"
equation "d121_1 = driver_length"
equation "d129_1 = -pwr_slack_outside"
equation "d130_1 = pwr_slack"
equation "d131_1 = pwr_width"
equation "d132_1 = ( pwr_length - pwr_interv * 4 ) / 2"
equation "d133_1 = pwr_width"
equation "d134_1 = pwr_interv"
equation "d137_1 = pwr_width"
equation "d138_1 = pwr_interv"
equation "d148_1 = elem_fix_spacer_height"
equation "d150_1 = elem_fix_spacer_height + pwr_z_offset"
equation "d153_1 = elem_fix_fillet"
equation "d158_1 = elem_fix_screw_hole_diam"
equation "d161_1 = elem_fix_screw_hole_diam"
equation "d164_1 = elem_fix_screw_hole_diam"
equation "d167_1 = elem_fix_screw_hole_diam"
equation "d170_1 = elem_fix_screw_hole_diam"
equation "d173_1 = elem_fix_screw_hole_diam"
equation "d176_1 = elem_fix_screw_hole_diam"
equation "d179_1 = elem_fix_screw_hole_diam"
equation "d182_1 = elem_fix_screw_hole_diam"
equation "d185_1 = elem_fix_screw_hole_diam"
equation "d188_1 = elem_fix_screw_hole_diam"
equation "d191_1 = elem_fix_screw_hole_diam"
equation "d194_1 = elem_fix_screw_hole_diam"
equation "d197_1 = elem_fix_screw_hole_diam"
equation "d200_1 = elem_fix_screw_hole_diam"
equation "d203_1 = elem_fix_screw_hole_diam"
equation "d206_1 = pwr_fix_screw_hole_diam"
equation "d209_1 = pwr_fix_screw_hole_diam"
equation "d212_1 = pwr_fix_screw_hole_diam"
equation "d215 = pwr_fix_screw_hole_diam"
equation "d217_1 = height + elem_fix_spacer_height"
equation "d218_1 = pwr_fix_screw_hole_diam"
equation "d220_1 = height + elem_fix_spacer_height"
equation "d221_1 = pwr_fix_screw_hole_diam"
equation "d223_1 = height + elem_fix_spacer_height"
equation "d224_1 = pwr_fix_screw_hole_diam"
equation "d226_1 = height + elem_fix_spacer_height"
equation "d227_1 = pwr_fix_screw_hole_diam"
equation "d230_1 = floor_spacer_size"
equation "d231_1 = floor_spacer_size"
equation "d232_1 = floor_spacer_size"
equation "d233_1 = floor_spacer_size"
equation "d234_1 = floor_spacer_size"
equation "d235_1 = floor_spacer_size"
equation "d237_1 = floor_spacer_size"
equation "d238_1 = floor_cut_length"
equation "d239_1 = floor_spacer_size"
equation "d240_1 = floor_spacer_size"
equation "d241_1 = floor_spacer_size"
equation "d242_1 = floor_spacer_size"
equation "d243_1 = floor_spacer_size"
equation "d244_1 = floor_spacer_size / 2"
equation "d245_1 = floor_spacer_size"
equation "d246_1 = floor_spacer_size / 2"
equation "d247_1 = floor_spacer_size"
equation "d248_1 = floor_spacer_size"
equation "d249_1 = floor_spacer_size"
equation "d250_1 = floor_spacer_size"
equation "d252_1 = floor_z_offset"
equation "d255_1 = floor_fix_fillet"
equation "d259_1 = floor_fix_fillet_add"
equation "d260_1 = height + elem_fix_spacer_height"
equation "d261_1 = elem_fix_screw_hole_diam"
equation "d263_1 = height + elem_fix_spacer_height"
equation "d264_1 = elem_fix_screw_hole_diam"
equation "d266_1 = height + elem_fix_spacer_height"
equation "d267_1 = elem_fix_screw_hole_diam"
equation "d269_1 = height + elem_fix_spacer_height"
equation "d270_1 = elem_fix_screw_hole_diam"
equation "d272_1 = height + elem_fix_spacer_height"
equation "d273_1 = elem_fix_screw_hole_diam"
equation "d275_1 = height + elem_fix_spacer_height"
equation "d276_1 = elem_fix_screw_hole_diam"
equation "d278_1 = height + elem_fix_spacer_height"
equation "d279 = elem_fix_screw_hole_diam"
equation "d281_1 = height + elem_fix_spacer_height"
equation "d282_1 = elem_fix_screw_hole_diam"
equation "d285_1 = width"
equation "d286_1 = length - ( batt_length + batt_wall * 2 )"
equation "d287_1 = floor_cut_width"
equation "d288_1 = floor_cut_length"
equation "d289_1 = height"
equation "d291_1 = floor_spacer_size"
equation "d292_1 = floor_spacer_size"
equation "d293_1 = floor_spacer_size"
equation "d294_1 = floor_spacer_size"
equation "d295_1 = floor_spacer_size"
equation "d296_1 = floor_spacer_size"
equation "d297_1 = floor_spacer_size"
equation "d298_1 = floor_spacer_size"
equation "d299_1 = floor_spacer_size"
equation "d300_1 = floor_spacer_size"
equation "d301_1 = floor_spacer_size"
equation "d302_1 = bms_length + bms_wall * 2"
equation "d303_1 = floor_spacer_size"
equation "d304_1 = floor_spacer_size / 2"
equation "d305_1 = floor_spacer_size"
equation "d306_1 = floor_spacer_size / 2"
equation "d307_1 = floor_spacer_size"
equation "d308_1 = floor_spacer_size"
equation "d310_1 = floor_fix_screw_ext_hole_diam"
equation "d311_1 = floor_fix_screw_ext_hole_diam"
equation "d312_1 = floor_fix_screw_ext_hole_diam"
equation "d313_1 = floor_fix_screw_ext_hole_diam"
equation "d314_1 = floor_fix_screw_ext_hole_diam"
equation "d315_1 = floor_fix_screw_ext_hole_diam"
equation "d316_1 = floor_fix_screw_ext_hole_diam"
equation "d317_1 = floor_fix_screw_ext_hole_diam"
equation "d326_1 = bms_width + bms_wall * 2"
equation "d327_1 = bms_wall"
equation "d328_1 = bms_thick + bms_wall * 2"
equation "d332_1 = -bms_wall"
equation "d335_1 = elem_fix_screw_hole_diam"
equation "d338_1 = elem_fix_screw_hole_diam"
equation "d341_1 = bms_fix_screw_ext_hole_diam"
equation "d344_1 = bms_fix_screw_ext_hole_diam"
equation "d348_1 = -slack_print"
equation "d350_1 = -slack_print"
equation "d352_1 = -slack_print"
equation "d354_1 = -slack_print"
equation "d356_1 = -slack_print"
equation "d358_1 = -slack_print"
equation "d360_1 = -slack_print"
equation "d362_1 = -slack_print"
equation "d364_1 = -slack_print"
equation "d370_1 = -batt_wall - slack_print"
equation "d371_1 = -slack_print"
equation "d373_1 = -batt_cover_height"
equation "d375_1 = batt_wall"
equation "d377_1 = batt_wall * 2"
equation "d378_1 = batt_wall"
equation "d379_1 = batt_wall"
equation "d380_1 = batt_wall"
equation "d381_1 = batt_wall * 2"
equation "d382_1 = batt_wall"
equation "d383_1 = batt_wall"
equation "d384_1 = batt_wall"
equation "d385_1 = elem_fix_screw_hole_diam"
equation "d386_1 = elem_fix_screw_hole_diam"
equation "d389_1 = batt_length + batt_wall * 2"
equation "d390_1 = batt_wall"
equation "d391_1 = batt_wall / 2"
equation "d392_1 = batt_wall"
equation "d393_1 = batt_wall / 2"
equation "d394_1 = batt_wall"
equation "d395_1 = elem_fix_screw_hole_diam"
equation "d399_1 = batt_cover_fix_screw_ext_hole_diam"
equation "d400_1 = batt_cover_fix_screw_ext_hole_diam"
equation "d401_1 = batt_cover_fix_screw_ext_hole_diam"
equation "d406_1 = batt_wall"
equation "d407_1 = batt_wall + slack_print"
equation "d408_1 = batt_wall + slack_print"
equation "d409_1 = batt_wall"
equation "d410_1 = batt_wall"
equation "d420_1 = arduino_length"
equation "d421_1 = arduino_width"
equation "d428_1 = elem_fix_spacer_diam"
equation "d429_1 = elem_fix_spacer_diam"
equation "d430_1 = arduino_length"
equation "d436 = elem_fix_spacer_height"
equation "d443_1 = elem_fix_screw_hole_diam"
equation "d446_1 = elem_fix_screw_hole_diam"
equation "d449_1 = elem_fix_screw_hole_diam"
equation "d452_1 = elem_fix_screw_hole_diam"
equation "d455_1 = elem_fix_fillet"
equation "d466_1 = -elem_fix_head_height"
equation "d468_1 = elem_fix_head_diam"
equation "d469_1 = elem_fix_head_diam"
equation "d470_1 = elem_fix_head_diam"
equation "d471_1 = elem_fix_head_diam"
equation "d472_1 = -elem_fix_head_height"
equation "d474_1 = elem_fix_head_diam"
equation "d475_1 = -elem_fix_head_height"
equation "d477_1 = elem_fix_head_diam"
equation "d478_1 = elem_fix_head_diam"
equation "d479_1 = elem_fix_head_diam"
equation "d480_1 = elem_fix_head_diam"
equation "d481_1 = elem_fix_head_diam"
equation "d482_1 = elem_fix_head_diam"
equation "d483_1 = elem_fix_head_diam"
equation "d484_1 = elem_fix_head_diam"
equation "d485_1 = elem_fix_head_diam"
equation "d486_1 = elem_fix_head_diam"
equation "d487_1 = elem_fix_head_diam"
equation "d488_1 = elem_fix_head_diam"
equation "d489_1 = elem_fix_head_diam"
equation "d490_1 = -elem_fix_head_height"
equation "d493_1 = elem_fix_fillet"
equation "d495_1 = elem_fix_fillet"
equation "width = 200 mm"
equation "length = 180 mm"
equation "height = 5 mm"
equation "screw_hole_diam = 4 mm"
equation "screw_head_diam = 7.5 mm"
equation "screw_offset = 10 mm"
equation "batt_width = 170 mm"
equation "batt_length = 30 mm"
equation "batt_height = 70 mm"
equation "batt_wall = 5 mm"
equation "batt_pwr_height = 10 mm"
equation "batt_cel_length = 4 mm"
equation "batt_cel_height = batt_height - batt_pwr_height - 5 mm"
equation "driver_width = 43 mm"
equation "driver_length = 76 mm"
equation "driver_screw_offset = 7.5 mm / 2"
equation "driver_space = 3 mm"
equation "elem_fix_screw_hole_diam = 2 mm + slack_print"
equation "elem_fix_spacer_diam = 6 mm"
equation "elem_fix_spacer_height = 5 mm"
equation "elem_fix_fillet = 2 mm"
equation "driver_fix_fillet = 1 mm"
equation "bms_width = 59 mm"
equation "bms_length = 20 mm"
equation "bms_thick = 1.5 mm"
equation "bms_wall = 5 mm"
equation "bms_bottom_slack = 3 mm"
equation "pwr_width = 27 mm"
equation "pwr_interv = 11.5 mm"
equation "pwr_length = pwr_interv * 4 + pwr_interv"
equation "pwr_z_offset = 20 mm"
equation "pwr_slack = 2.5 mm + 5 mm"
equation "pwr_slack_outside = 5 mm"
equation "pwr_fix_screw_hole_diam = elem_fix_screw_hole_diam"
equation "floor_spacer_size = 6 mm"
equation "floor_cut_length = length - ( batt_length + batt_wall * 2 ) - driver_length"
equation "floor_z_offset = batt_height / 2 - height"
equation "floor_fix_fillet = elem_fix_fillet"
equation "floor_fix_fillet_add = 5 mm"
equation "floor_cut_width = ( ( batt_width + batt_wall * 2 ) / 2 - ( bms_width + bms_wall * 2 ) / 2 ) + width - ( batt_wall * 2 + batt_width )"
equation "floor_fix_screw_ext_hole_diam = 3 mm + slack_print"
equation "bms_fix_screw_ext_hole_diam = floor_fix_screw_ext_hole_diam - 0.5 mm"
equation "slack_print = 0.5 mm"
equation "batt_cover_height = batt_wall * 3"
equation "batt_cover_fix_screw_ext_hole_diam = floor_fix_screw_ext_hole_diam"
equation "arduino_length = 57 mm"
equation "arduino_width = 113 mm"
equation "elem_fix_head_diam = 6.5 mm"
equation "elem_fix_head_height = 2.5 mm"
named bodies: "baseplate", "floor", "bms_fixate", "batt_cover"
